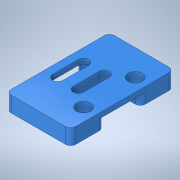
# Autodesk Inventor part: Small_Belt_Clamp
Saved by Autodesk Inventor 2021 (Build 250183000, 183)
## iProperties
Created: 2021-02-03
Part Number: Small_Belt_Clamp
Material: Generic
Document SubType Name: Modeling
Designer: Jorian Brusind
Density: 1 g/cm^3
Appearance: Cyan
Author: Jorian Brusind
Autodesk Inventor part; units mm, degrees
ref_plane "YZ Plane" through (0, 0, 0) normal (1, 0, 0) x (0, 1, 0)
ref_plane "XZ Plane" through (0, 0, 0) normal (0, 1, 0) x (-1, 0, 0)
ref_plane "XY Plane" through (0, 0, 0) normal (0, 0, 1) x (1, 0, 0)
sketch "Sketch1" plane through (0, 0, 0) normal (0, 1, 0) x (-1, 0, 0)
  line L0 (0, 0) -> (10, 0)
  line L1 (10, 0) -> (10, -40)
  line L2 (10, -40) -> (0, -40)
  line L3 (0, -40) -> (0, 0)
  line L4 (10, 0) -> (25, 0)
  line L5 (25, 0) -> (25, -40)
  line L6 (25, -40) -> (10, -40)
  line L7 (10, -40) -> (10, 0)
  dimension "d0" = 10
  dimension "d1" = 40
  dimension "d2" = 15
  dimension "d3" = 40
  constraints: 16 end point, 4 parallel, 2 horizontal, 2 perpendicular
  measures "d0" distance of L1.end L2.end
  measures "d1" distance of L0.end L1.end
  measures "d2" distance of L5.end L6.end
  measures "d3" distance of L4.end L5.end
extrude "Extrusion1" add sketch "Sketch1" along normal blind 6
sketch "Sketch2" plane through (0, 6, 0) normal (0, 1, 0) x (1, 0, 0)
  circle A0 centre (-5, 10) radius 2.75
  line L0 (0, 0) -> (0, 40) projected
  line L1 (-25, 0) -> (0, 0) projected
  circle A1 centre (-5, 30) radius 2.75
  line L2 (-25, 40) -> (-25, 0) projected
  line L3 (-25, 20) -> (-20, 20)
  line L4 (-20, 20) -> (-12, 20)
  line L5 (-20, 15) -> (-20, 25) construction
  line L6 (-18, 15) -> (-18, 25)
  line L7 (-22, 25) -> (-22, 15)
  arc A2 (-22, 15) -> (-18, 15) centre (-20, 15) ccw
  arc A3 (-18, 25) -> (-22, 25) centre (-20, 25) ccw
  line L8 (-12, 15) -> (-12, 25) construction
  line L9 (-10, 15) -> (-10, 25)
  line L10 (-14, 25) -> (-14, 15)
  arc A4 (-14, 15) -> (-10, 15) centre (-12, 15) ccw
  arc A5 (-10, 25) -> (-14, 25) centre (-12, 25) ccw
  line L11 (-12, 20) -> (-2, 20) construction
  dimension "d6" = 5.5
  dimension "d7" = 5
  dimension "d8" = 10
  dimension "d9" = 5.5
  dimension "d10" = 5
  dimension "d11" = 20
  dimension "d12" = 5
  dimension "d13" = 8
  dimension "d14" = 5
  dimension "d15" = 4
  dimension "d16" = 5
  dimension "d17" = 90
  dimension "d18" = 4
  constraints: 22 end point, 8 point on circle, 8 tangent, 6 centre point, 3 midpoint, 3 parallel, 2 horizontal, 2 perpendicular, 1 point on line
  measures "d6" diameter of A0
  measures "d7" distance from line of L0 A0.centre
  measures "d8" distance from line of L1 A0.centre
  measures "d9" diameter of A1
  measures "d10" distance from line of L0 A1.centre
  measures "d11" distance of A0.centre A1.centre
  measures "d12" distance of L3.start L3.end
  measures "d13" distance of L3.end L4.end
  measures "d14" distance of L3.end L5.end
  measures "d15" diameter of A3
  measures "d16" distance of L4.end L8.end
  measures "d17" angle of L11 L8
  measures "d18" diameter of A5
extrude "Extrusion2" cut sketch "Sketch2" against normal up to next
fillet "Fillet1" radius 2 4 edges at (0, 3, 0) (-25, 3, 0) (0, 3, -40) (-25, 3, -40)
sketch "Sketch3" plane through (-25, 0, -38) normal (-1, 0, 0) x (0, 0, 1)
  line L0 (23, 6) -> (13, 6) projected
  line L1 (18, 6) -> (25, 6)
  line L2 (36, 0) -> (0, 0) projected
  line L3 (18, 0) -> (25, 0)
  line L4 (25, 0) -> (11, 0)
  line L5 (11, 0) -> (11, 4)
  line L6 (11, 4) -> (25, 4)
  line L7 (25, 4) -> (25, 0)
  point P0 (38, 0)
  point P1 (11, 0)
  dimension "d22" = 7
  dimension "d23" = 7
  dimension "d24" = 14
  dimension "d25" = 4
  constraints: 12 end point, 2 midpoint, 2 parallel, 1 collinear, 1 horizontal, 1 perpendicular, 1 point on line
  measures "d22" distance of L1.start L1.end
  measures "d23" distance of L3.start L3.end
  measures "d24" distance of L5.end L6.end
  measures "d25" distance of L4.end L5.end
extrude "Extrusion3" cut sketch "Sketch3" against normal blind 8
sketch "Sketch4" plane through (0, 0, 0) normal (0, -1, 0) x (1, 0, 0)
  line L0 (-14, -25) -> (-14, -15) projected
  line L1 (-14, -20) -> (-14, -13)
  line L2 (-14, -20) -> (-7, -20) construction
  line L3 (-14, -13) -> (0, -13)
  line L4 (0, -13) -> (0, -27)
  line L5 (0, -27) -> (-14, -27)
  line L6 (-14, -27) -> (-14, -13)
  point P0 (0, 0)
  dimension "d28" = 7
  dimension "d29" = 90
  dimension "d30" = 14
  dimension "d31" = 14
  constraints: 12 end point, 2 horizontal, 2 parallel, 2 perpendicular, 1 midpoint, 1 vertical
  measures "d28" distance of L1.start L1.end
  measures "d29" angle of L2 L1
  measures "d30" distance of L4.end L5.end
  measures "d31" distance of L3.end L4.end
extrude "Extrusion4" cut sketch "Sketch4" against normal blind 4
fillet "Fillet2" radius 2 4 edges at (-14, 2, -13) (-17, 2, -13) (-14, 2, -27) (-17, 2, -27)
fillet "Fillet3" radius 2 4 edges at (-25, 2, -27) (-25, 2, -13) (0, 2, -27) (0, 2, -13)
body "Solid1"
